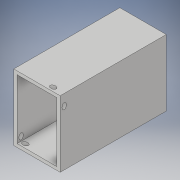
# Autodesk Inventor part: cage
Saved by Autodesk Inventor 2019 (Build 230136000, 136)
## iProperties
Created: 2021-05-02
Part Number: cage
Material: Generisch
Document SubType Name: Modeling
Designer: Michael Hohenstein
Density: 1 g/cm^3
Appearance: Vorgabe
Author: Michael Hohenstein
Autodesk Inventor part; units mm, degrees
ref_plane "YZ Plane" through (0, 0, 0) normal (1, 0, 0) x (0, 1, 0)
ref_plane "XZ Plane" through (0, 0, 0) normal (0, 1, 0) x (-1, 0, 0)
ref_plane "XY Plane" through (0, 0, 0) normal (0, 0, 1) x (1, 0, 0)
sketch "Skizze1" plane through (0, 0, 0) normal (0, 0, 1) x (1, 0, 0)
  line L0 (-15, -22.5) -> (15, -22.5)
  line L1 (15, -22.5) -> (15, 22.5)
  line L2 (15, 22.5) -> (-15, 22.5)
  line L3 (-15, 22.5) -> (-15, -22.5)
  line L4 (17.5, 25) -> (17.5, -25)
  line L5 (17.5, -25) -> (-17.5, -25)
  line L6 (-17.5, -25) -> (-17.5, 25)
  line L7 (-17.5, 25) -> (17.5, 25)
  point P0 (0, 0)
  point P1 (0, 22.5)
  point P2 (15, 0)
  dimension "d0" = 45
  dimension "d1" = 30
  dimension "d2" = 2.5
  constraints: 16 end point, 4 parallel, 2 midpoint, 2 perpendicular, 1 horizontal, 1 horizontal alignment, 1 vertical alignment, 3 other
  measures "d0" distance of L0.end L1.end
  measures "d1" distance of L1.end L2.end
  measures "d2" distance between parallel lines of L1 L4
extrude "Extrusion1" add sketch "Skizze1" against normal blind 2.5 contours L3 L2 L1 L0 | L4 L5 L6 L7
extrude "Extrusion2" add sketch "Skizze1" along normal blind 77.5
sketch "Skizze2" plane through (0, 0, -2.5) normal (0, 0, -1) x (-1, 0, 0)
  circle A0 centre (0, 0) radius 1.5
  dimension "d7" = 3
  constraints: 1 centre point, 1 coincident
  measures "d7" diameter of A0
extrude "Extrusion3" cut sketch "Skizze2" against normal up to surface (2.5 mm away)
sketch "Skizze3" plane through (0, 0, 77.5) normal (0, 0, 1) x (1, 0, 0)
  line L0 (5.0147, 25) -> (13.5, 25)
  line L1 (13.5, 25) -> (9.2574, 29.2426)
  line L2 (9.2574, 29.2426) -> (5.0147, 25)
  line L3 (17.5, 21) -> (17.5, 12.5147)
  line L4 (17.5, 12.5147) -> (21.7426, 16.7574)
  line L5 (21.7426, 16.7574) -> (17.5, 21)
  line L6 (17.5, 25) -> (-17.5, 25) projected
  line L7 (17.5, -25) -> (17.5, 25) projected
  line L8 (7.136, 27.1213) -> (19.6213, 14.636) construction
  line L9 (-17.5, -12.5147) -> (-17.5, -21)
  line L10 (-17.5, -21) -> (-21.7426, -16.7574)
  line L11 (-21.7426, -16.7574) -> (-17.5, -12.5147)
  line L12 (-13.5, -25) -> (-5.0147, -25)
  line L13 (-5.0147, -25) -> (-9.2574, -29.2426)
  line L14 (-9.2574, -29.2426) -> (-13.5, -25)
  line L15 (-17.5, 25) -> (-17.5, -25) projected
  line L16 (-17.5, -25) -> (17.5, -25) projected
  line L17 (-19.6213, -14.636) -> (-7.136, -27.1213) construction
  point P0 (0, 0)
  dimension "d11" = 6
  dimension "d17" = 4
  dimension "d18" = 4
  constraints: 28 end point, 10 equal length, 4 midpoint, 4 point on line, 2 horizontal, 2 perpendicular, 2 vertical, 1 parallel
  measures "d11" distance of L0.end L1.end
  measures "d17" distance of L3.start L6.start
  measures "d18" distance of L9.end L15.end
extrude "Extrusion4" add sketch "Skizze3" against normal blind 6 contours L2 L1 L0 | L9 L10 L11 | L5 L4 L3 | L12 L13 L14
sketch "Skizze4" plane through (9.2574, 29.2426, 71.5) normal (-0.7071, 0.7071, 0) x (-0.7071, -0.7071, 0)
  line L0 (0, 0) -> (6, 0) construction
  line L1 (6, 6) -> (0, 6) construction
  line L2 (0, 0) -> (6, 0) construction
  line L3 (6, 0) -> (6, 6) construction
  line L4 (6, 6) -> (0, 6) construction
  line L5 (0, 6) -> (0, 0) construction
  circle A0 centre (3, 3) radius 1.65
  point P0 (27.2236, -71.5)
  point P1 (3, 6)
  point P2 (0, 3)
  dimension "d14" = 3.3
  constraints: 8 end point, 2 midpoint, 2 parallel, 1 centre point, 1 horizontal, 1 horizontal alignment, 1 perpendicular, 1 vertical alignment
  measures "d14" diameter of A0
extrude "Extrusion5" cut sketch "Skizze4" against normal up to surface (17.6569 mm away)
sketch "Skizze5" plane through (-17.5, -12.5147, 71.5) normal (-0.7071, 0.7071, 0) x (-0.7071, -0.7071, 0)
  line L0 (0, 0) -> (6, 0) construction
  line L1 (0, 6) -> (6, 6) construction
  line L2 (0, 0) -> (6, 0) construction
  line L3 (6, 0) -> (6, 6) construction
  line L4 (6, 6) -> (0, 6) construction
  line L5 (0, 6) -> (0, 0) construction
  circle A0 centre (3, 3) radius 1.65
  point P0 (-21.2236, -71.5)
  point P1 (3, 6)
  point P2 (0, 3)
  dimension "d19" = 3.3
  constraints: 8 end point, 2 midpoint, 2 parallel, 1 centre point, 1 horizontal, 1 horizontal alignment, 1 perpendicular, 1 vertical alignment
  measures "d19" diameter of A0
extrude "Extrusion6" cut sketch "Skizze5" against normal up to surface (17.6569 mm away)
sketch "Skizze6" plane through (0, 0, 77.5) normal (0, 0, 1) x (1, 0, 0)
  line L0 (-21.7426, -29.2426) -> (21.7426, -29.2426)
  line L1 (21.7426, -29.2426) -> (21.7426, 29.2426)
  line L2 (21.7426, 29.2426) -> (-21.7426, 29.2426)
  line L3 (-21.7426, 29.2426) -> (-21.7426, -29.2426)
  line L4 (17.5, 25) -> (13.5, 25) projected
  line L5 (17.5, 25) -> (-17.5, 25)
  line L6 (-17.5, 25) -> (-17.5, -25)
  line L7 (-17.5, -25) -> (17.5, -25)
  line L8 (17.5, -25) -> (17.5, 25)
  point P0 (0, 0)
  point P1 (9.2574, 29.2426)
  point P2 (21.7426, 16.7574)
  point P3 (-9.2574, -29.2426)
  point P4 (-21.7426, -16.7574)
  constraints: 16 end point, 4 parallel, 4 point on line, 2 horizontal, 2 perpendicular
extrude "Extrusion7" cut sketch "Skizze6" against normal up to surface (6 mm away)
equation "\"d18\" = d17"
